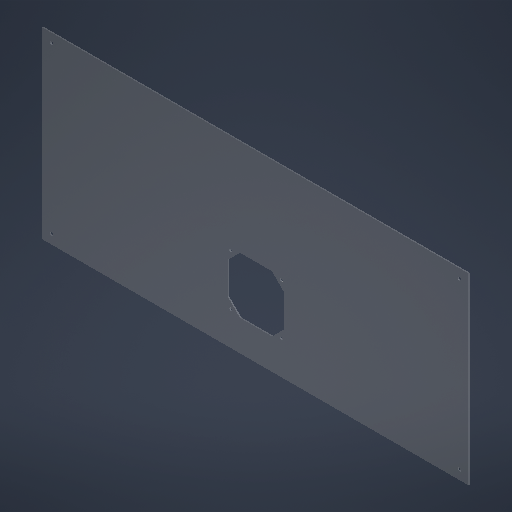
# Autodesk Inventor part: PlaqueVentilo2
Saved by Autodesk Inventor 2026.2 (Build 302298010, 298A)
## iProperties
Part Number: PlaqueVentilo2
Material: Générique
Document SubType Name: Modélisation
Designer: quent
Appearance: Transparent - Clair
Author: quent
Autodesk Inventor part; units mm, degrees
ref_plane "Plan YZ" through (0, 0, 0) normal (1, 0, 0) x (0, 1, 0)
ref_plane "Plan XZ" through (0, 0, 0) normal (0, 1, 0) x (-1, 0, 0)
ref_plane "Plan XY" through (0, 0, 0) normal (0, 0, 1) x (1, 0, 0)
sketch "Esquisse1" plane through (0, 0, 0) normal (0, 0, 1) x (1, 0, 0)
  line L0 (-198.5648, -151.8074) -> (495.4352, -151.8074)
  line L1 (495.4352, -151.8074) -> (495.4352, 147.1926)
  line L2 (495.4352, 147.1926) -> (-198.5648, 147.1926)
  line L3 (-198.5648, 147.1926) -> (-198.5648, -151.8074)
  line L4 (-198.5648, -151.8074) -> (495.4352, 147.1926) construction
  line L5 (-186.0648, -139.3074) -> (482.9352, -139.3074)
  line L6 (482.9352, -139.3074) -> (482.9352, 134.6926)
  line L7 (482.9352, 134.6926) -> (-186.0648, 134.6926)
  line L8 (-186.0648, 134.6926) -> (-186.0648, -139.3074)
  line L9 (-186.0648, -139.3074) -> (482.9352, 134.6926) construction
  circle A0 centre (-183.5648, 132.1926) radius 2.5
  circle A1 centre (-183.5648, -136.8074) radius 2.5
  circle A2 centre (480.4352, -136.8074) radius 2.5
  circle A3 centre (480.4352, 132.1926) radius 2.5
  line L10 (123.4352, -9.8074) -> (175.4352, -9.8074)
  line L11 (195.4352, -29.8074) -> (195.4352, -81.8074)
  line L12 (175.4352, -101.8074) -> (123.4352, -101.8074)
  line L13 (103.4352, -81.8074) -> (103.4352, -29.8074)
  line L14 (103.4352, -9.8074) -> (195.4352, -101.8074) construction
  line L15 (195.4352, -9.8074) -> (103.4352, -101.8074) construction
  line L16 (123.4352, -9.8074) -> (103.4352, -29.8074)
  line L17 (103.4352, -81.8074) -> (123.4352, -101.8074)
  line L18 (175.4352, -101.8074) -> (195.4352, -81.8074)
  line L19 (195.4352, -29.8074) -> (175.4352, -9.8074)
  circle A4 centre (108.1852, -14.5574) radius 2.2
  circle A5 centre (190.6852, -14.5574) radius 2.2
  circle A6 centre (190.6852, -97.0574) radius 2.2
  circle A7 centre (108.1852, -97.0574) radius 2.2
  point P0 (0, 0)
  point P1 (148.4352, -2.3074)
  point P2 (149.4352, -55.8074)
  point P3 (-186.0648, -136.8074)
  point P4 (-183.5648, -139.3074)
  point P5 (480.4352, -139.3074)
  point P6 (482.9352, -136.8074)
  point P7 (482.9352, 132.1926)
  point P8 (480.4352, 134.6926)
  point P9 (-186.0648, 132.1926)
  point P10 (-183.5648, 134.6926)
  dimension "d0" = 694
  dimension "d1" = 299
  dimension "d2" = 12.5
  dimension "d3" = 12.5
  dimension "d4" = 5
  dimension "d5" = 5
  dimension "d6" = 5
  dimension "d7" = 5
  dimension "d8" = 92
  dimension "d9" = 92
  dimension "d10" = 50
  dimension "d11" = 300
  dimension "d12" = 20
  dimension "d13" = 20
  dimension "d14" = 20
  dimension "d15" = 20
  dimension "d16" = 20
  dimension "d17" = 20
  dimension "d18" = 20
  dimension "d19" = 20
  dimension "d20" = 4.4
  dimension "d21" = 4.4
  dimension "d22" = 4.4
  dimension "d23" = 4.4
  dimension "d24" = 4.75
  dimension "d25" = 4.75
  constraints: 40 end point, 19 point on line, 8 centre point, 8 tangent, 6 parallel, 4 midpoint, 3 horizontal, 3 perpendicular
  measures "d0" distance of L2.end L4.end
  measures "d1" distance of L4.end L0.end
  measures "d2" distance between parallel lines of L2 L7
  measures "d3" distance between parallel lines of L1 L6
  measures "d4" diameter of A0
  measures "d5" diameter of A1
  measures "d6" diameter of A2
  measures "d7" diameter of A3
  measures "d8" distance of L14.end L15.end
  measures "d9" distance of L15.start L14.end
  measures "d10" distance between parallel lines of L0 L12
  measures "d11" distance between parallel lines of L1 L11
  measures "d12" distance of L16.start point (103.435, -9.807)
  measures "d13" distance of L13.end point (103.435, -9.807)
  measures "d14" distance of L13.start point (103.435, -101.807)
  measures "d15" distance of L17.end point (103.435, -101.807)
  measures "d16" distance of L12.start point (195.435, -101.807)
  measures "d17" distance of L18.end point (195.435, -101.807)
  measures "d18" distance of L11.start point (195.435, -9.807)
  measures "d19" distance of L10.end point (195.435, -9.807)
  measures "d20" diameter of A4
  measures "d21" diameter of A5
  measures "d22" diameter of A6
  measures "d23" diameter of A7
  measures "d24" horizontal distance of L14.start A4.centre
  measures "d25" horizontal distance of L14.start A4.centre
extrude "Extrusion1" add sketch "Esquisse1" along normal blind 2 contours L3 L2 L1 L0 | A1 L8 A0 L7 A3 L6 A2 L5
equation "\"d13\" = d12"
equation "\"d14\" = d12"
equation "\"d15\" = d14"
equation "\"d16\" = d12"
equation "\"d17\" = d16"
equation "\"d18\" = d12"
equation "\"d19\" = d18"
